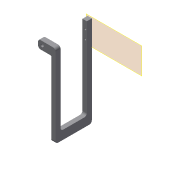
# Autodesk Inventor part: 06_Fluorescence_Arm
Saved by Autodesk Inventor 2019.4 (Build 234330000, 330)
## iProperties
Created: 2021-02-17
Part Number: 06_Fluorescence_Arm
Material: Generic
Document SubType Name: Modeling
Designer: diederichbenedict
Density: 1 g/cm^3
Appearance: Default
Author: diederichbenedict
Autodesk Inventor part; units mm, degrees
ref_plane "YZ Plane" through (0, 0, 0) normal (1, 0, 0) x (0, 1, 0)
ref_plane "XZ Plane" through (0, 0, 0) normal (0, 1, 0) x (-1, 0, 0)
ref_plane "XY Plane" through (0, 0, 0) normal (0, 0, 1) x (1, 0, 0)
ref_plane "Work Plane1" through (0, 0, 0) normal (0, 0, 1) x (1, 0, 0)
sketch "Sketch1" plane through (0, 0, 0) normal (0, 0, 1) x (1, 0, 0)
  circle A0 centre (-15.5, 7) radius 1.45 projected
  circle A1 centre (-15.5, -7) radius 1.45 projected
  line L0 (63, 19) -> (63, -19) projected
  circle A2 centre (56, -16.5) radius 1.45 projected
  circle A3 centre (60.5, 16.5) radius 1.45 projected
  circle A4 centre (-15.5, 7) radius 1.45 projected
  circle A5 centre (-15.5, -7) radius 1.45 projected
  circle A6 centre (60.5, -16.5) radius 1.45 projected
  circle A7 centre (56, 16.5) radius 1.45 projected
  circle A8 centre (10, 10) radius 1.75 projected
  circle A9 centre (-10, -10) radius 1.75 projected
  circle A10 centre (10, -10) radius 1.75 projected
  line L1 (31.25, -14.25) -> (31.25, 14.25) projected
  line L2 (31.25, 14.25) -> (59.75, 14.25) projected
  line L3 (59.75, 14.25) -> (59.75, -14.25) projected
  line L4 (59.75, -14.25) -> (31.25, -14.25) projected
  circle A11 centre (-10, 10) radius 1.75 projected
  line L5 (-18, 19) -> (63, 19) projected
  line L6 (-18, -19) -> (-18, 19) projected
  line L7 (63, -19) -> (-18, -19) projected
  line L8 (63, 19) -> (63, -19) projected
  line L9 (-18, 19) -> (-13, 19)
  line L10 (-13, 19) -> (-13, -126)
  line L11 (-13, -126) -> (-18, -126)
  line L12 (-18, -126) -> (-18, 19)
  point P0 (0, 0)
  dimension "d0" = 5
  dimension "d1" = 145
  constraints: 8 end point, 2 parallel, 1 horizontal, 1 perpendicular
  measures "d0" distance of L10.end L11.end
  measures "d1" distance of L9.end L10.end
extrude "Extrusion1" add sketch "Sketch1" along normal blind 8 contours L10 L7 L6 L5 | L10 L11 L12 L7
sketch "Sketch2" plane through (0, 0, 8) normal (0, 0, 1) x (1, 0, 0)
  circle A0 centre (-15.5, -7) radius 1.45 projected
  circle A1 centre (-15.5, 7) radius 1.45 projected
  line L0 (-13, 19) -> (-18, 19) projected
  line L1 (-18, 19) -> (-18, -126) projected
  line L2 (-18, -126) -> (-13, -126) projected
  line L3 (-13, -126) -> (-13, 19) projected
  line L4 (-18, 19) -> (-18, -126) projected
  line L5 (-13, -126) -> (-13, 19) projected
  line L6 (-18, -126) -> (-13, -126)
  line L7 (-13, -126) -> (-13, -112)
  line L8 (-13, -112) -> (-18, -112)
  line L9 (-18, -112) -> (-18, -126)
  point P0 (0, 0)
  dimension "d4" = 14
  constraints: 8 end point, 2 parallel, 1 horizontal, 1 perpendicular, 1 point on line
  measures "d4" distance of L7.end L6.end
extrude "Extrusion2" add sketch "Sketch2" along normal blind 50 contours L3 L2 L1 L8
sketch "Sketch3" plane through (0, 0, 58) normal (0, 0, 1) x (1, 0, 0)
  circle A0 centre (-34.5766, 0) radius 2.4142 projected
  line L0 (-18, -126) -> (-13, -126) projected
  line L1 (-13, -126) -> (-13, -112) projected
  line L2 (-13, -112) -> (-18, -112) projected
  line L3 (-18, -112) -> (-18, -126) projected
  line L4 (-13, 19) -> (-13, -126) projected
  line L5 (-18, -112) -> (-13, -112)
  line L6 (-13, -112) -> (-13, 6)
  line L7 (-13, 6) -> (-18, 6)
  line L8 (-18, 6) -> (-18, -112)
  line L9 (-18, 6) -> (-41, 6)
  line L10 (-41, 6) -> (-41, -7)
  line L11 (-41, -7) -> (-18, -7)
  line L12 (-18, -7) -> (-18, 6)
  circle A1 centre (-34.5766, 0) radius 2.5
  point P0 (0, 0)
  dimension "d7" = 118
  dimension "d8" = 23
  dimension "d9" = 13
  dimension "d10" = 5
  constraints: 16 end point, 4 parallel, 2 horizontal, 2 perpendicular, 1 centre point, 1 coincident, 1 point on line
  measures "d7" distance of L6.end L5.end
  measures "d8" distance of L11.end L10.end
  measures "d9" distance of L10.end L9.end
  measures "d10" diameter of A1
extrude "Extrusion3" add sketch "Sketch3" against normal blind 8 contours L3 L2 L1 L0 | L8 L7 L4 L2 | L11 L10 L9 L8
fillet "Fillet1" radius 4 8 edges at (-15.5, -112, 50) (-15.5, -112, 8) (-15.5, -126, 58) (-15.5, -126, 0) (-18, -7, 54) (-13, 6, 54) (-41, 6, 54) (-41, -7, 54)
sketch "Sketch4" plane through (-18, 19, 0) normal (-1, 0, 0) x (0, 0, 1)
  line L0 (50, -30) -> (58, -30) projected
  line L1 (50, -127) -> (50, -30) projected
  arc A0 (46, -131) -> (50, -127) centre (46, -127) ccw projected
  line L2 (12, -131) -> (46, -131) projected
  arc A1 (8, -127) -> (12, -131) centre (12, -127) ccw projected
  line L3 (8, 0) -> (8, -127) projected
  line L4 (0, 0) -> (8, 0) projected
  line L5 (0, -141) -> (0, 0) projected
  arc A2 (0, -141) -> (4, -145) centre (4, -141) ccw projected
  line L6 (4, -145) -> (54, -145) projected
  arc A3 (54, -145) -> (58, -141) centre (54, -141) ccw projected
  line L7 (58, -141) -> (58, -30) projected
  line L8 (50, -26) -> (50, -30) projected
  line L9 (50, -30) -> (58, -30) projected
  line L10 (58, -30) -> (58, -26) projected
  line L11 (58, -26) -> (50, -26) projected
  point P0 (0, -19)
extrude "Extrusion4" add sketch "Sketch4" along normal blind 2
body "Solid1"
